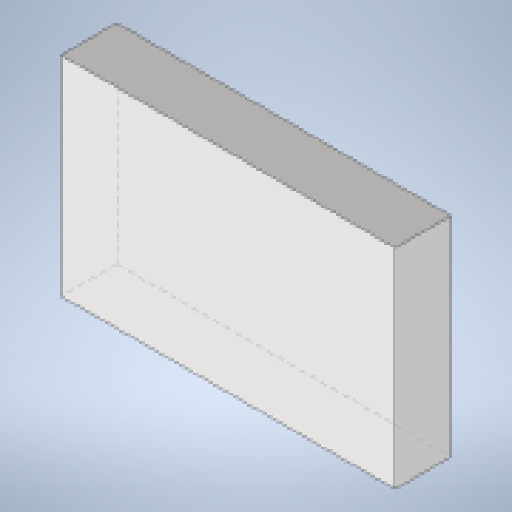
# Autodesk Inventor part: Battery
Saved by Autodesk Inventor 2024 (Build 280153000, 153)
## iProperties
Created: 2023-11-10
Part Number: Battery
Material: Generic
Document SubType Name: Modeling
Designer: jevan
Density: 1 g/cm^3
Appearance: Default
Author: jevan
Autodesk Inventor part; units mm, degrees
ref_plane "YZ Plane" through (0, 0, 0) normal (1, 0, 0) x (0, 1, 0)
ref_plane "XZ Plane" through (0, 0, 0) normal (0, 1, 0) x (-1, 0, 0)
ref_plane "XY Plane" through (0, 0, 0) normal (0, 0, 1) x (1, 0, 0)
sketch "Sketch1" plane through (0, 0, 0) normal (0, 0, 1) x (1, 0, 0)
  line L0 (-21.2741, -15.629) -> (-21.2741, 14.371)
  line L1 (-21.2741, 14.371) -> (26.7259, 14.371)
  line L2 (26.7259, 14.371) -> (26.7259, -15.629)
  line L3 (26.7259, -15.629) -> (-21.2741, -15.629)
  point P0 (0, 0)
  dimension "d3" = 30
  dimension "d4" = 48
  constraints: 8 end point, 2 parallel, 1 horizontal, 1 perpendicular
  measures "d3" distance of L0.start L0.end
  measures "d4" distance of L0.end L1.end
extrude "Extrusion1" add sketch "Sketch1" along normal blind 8
fillet "Fillet1" radius 2 10 edges at (2.7259, 14.371, 8) (2.7259, 14.371, 0) (2.7259, -15.629, 8) (2.7259, -15.629, 0) (26.7259, -0.629, 8) (26.7259, -0.629, 0) (-21.2741, 14.371, 4) (-21.2741, -0.629, 0) (-21.2741, -0.629, 8) (-21.2741, -15.629, 4)
body "Solid1"
